Autodesk Inventor part; units mm, degrees
note: some values were not read from the file. Chosen so that the rebuilt part matches the saved one: direction of "Hole2".
(part 17 of 18)
  line L1457 (-0.7456, -14.7218) -> (0.7544, -14.7219)
  line L1458 (0.7544, -14.7219) -> (0.7543, -15.7175)
  line L1459 (0.7543, -15.7175) -> (-0.7457, -15.7174)
  line L1460 (-0.7457, -15.7174) -> (-0.7456, -14.7218)
  line L1461 (0.7544, -14.7219) -> (0.6938, -14.8147)
  line L1462 (-0.7456, -14.7218) -> (-0.6851, -14.8146)
  line L1463 (-0.7457, -15.7174) -> (-0.6885, -15.691)
  line L1464 (0.7543, -15.7175) -> (0.6971, -15.6911)
  line L1465 (3.62, -17.1773) -> (3.8191, -17.1584)
  line L1466 (3.6201, -17.1773) -> (3.62, -17.1773)
  line L1467 (3.8426, -17.4073) -> (3.8427, -17.4073)
  line L1468 (3.8191, -17.1584) -> (3.8426, -17.4073)
  line L1469 (3.7248, -16.1629) -> (3.5257, -16.1817)
  line L1470 (3.7012, -15.914) -> (3.7248, -16.1629)
  line L1471 (3.62, -17.1773) -> (3.5257, -16.1817)
  line L1472 (3.7012, -15.914) -> (5.5927, -15.7349)
  line L1473 (5.7342, -17.2282) -> (3.8426, -17.4073)
  line L1474 (5.8154, -15.9649) -> (5.9097, -16.9604)
  line L1475 (5.5927, -15.7349) -> (5.5928, -15.7349)
  line L1476 (5.8154, -15.9649) -> (5.6163, -15.9837)
  line L1477 (5.6163, -15.9837) -> (5.5927, -15.7349)
  line L1478 (5.8155, -15.9649) -> (5.8154, -15.9649)
  line L1479 (5.7342, -17.2282) -> (5.7106, -16.9793)
  line L1480 (5.7106, -16.9793) -> (5.9097, -16.9604)
  line L1481 (5.9097, -16.9604) -> (5.9098, -16.9604)
  line L1482 (5.7106, -16.9793) -> (5.7107, -16.9793)
  line L1483 (5.7343, -17.2282) -> (5.7342, -17.2282)
  line L1484 (3.9239, -16.144) -> (5.4172, -16.0026)
  line L1485 (5.4172, -16.0026) -> (5.5115, -16.9981)
  line L1486 (5.5115, -16.9981) -> (4.0182, -17.1396)
  line L1487 (4.0182, -17.1396) -> (3.9239, -16.144)
  line L1488 (5.2584, -16.1948) -> (4.1161, -16.303)
  line L1489 (5.4172, -16.0026) -> (5.2584, -16.1948)
  line L1490 (3.9239, -16.144) -> (4.1161, -16.303)
  line L1491 (4.1161, -16.303) -> (4.1772, -16.9474)
  line L1492 (4.0182, -17.1396) -> (4.1772, -16.9474)
  line L1493 (4.1772, -16.9474) -> (5.3194, -16.8392)
  line L1494 (5.5115, -16.9981) -> (5.3194, -16.8392)
  line L1495 (5.3194, -16.8392) -> (5.2584, -16.1948)
  circle A30 centre (4.457, -16.5958) radius 0.1
  line L1496 (4.6323, -16.7299) -> (4.31, -16.7604)
  line L1497 (4.31, -16.7604) -> (4.2817, -16.4617)
  line L1498 (4.2817, -16.4617) -> (4.6041, -16.4312)
  line L1499 (4.6041, -16.4312) -> (4.6323, -16.7299)
  line L1500 (4.6041, -16.4312) -> (4.6324, -16.7299)
  line L1501 (-2.4972, -34.9673) -> (-2.4972, -34.7673)
  line L1502 (-2.4972, -34.7673) -> (-2.2472, -34.7673)
  line L1503 (-3.4972, -34.7672) -> (-3.4972, -34.9672)
  line L1504 (-3.7472, -34.7672) -> (-3.4972, -34.7672)
  line L1505 (-2.4972, -34.9673) -> (-3.4972, -34.9672)
  line L1506 (-3.7472, -34.7672) -> (-3.747, -32.8672)
  line L1507 (-2.247, -32.8673) -> (-2.2472, -34.7673)
  line L1508 (-3.497, -32.6672) -> (-2.497, -32.6673)
  line L1509 (-2.247, -32.8673) -> (-2.497, -32.8673)
  line L1510 (-2.497, -32.8673) -> (-2.497, -32.6673)
  line L1511 (-3.497, -32.6672) -> (-3.497, -32.8672)
  line L1512 (-3.497, -32.8672) -> (-3.747, -32.8672)
  line L1513 (-3.4971, -34.5672) -> (-3.497, -33.0672)
  line L1514 (-3.497, -33.0672) -> (-2.497, -33.0673)
  line L1515 (-2.497, -33.0673) -> (-2.4971, -34.5673)
  line L1516 (-2.4971, -34.5673) -> (-3.4971, -34.5672)
  line L1517 (-3.3207, -33.2435) -> (-3.3208, -34.3909)
  line L1518 (-3.497, -33.0672) -> (-3.3207, -33.2435)
  line L1519 (-3.4971, -34.5672) -> (-3.3208, -34.3909)
  line L1520 (-3.3208, -34.3909) -> (-2.6735, -34.3909)
  line L1521 (-2.4971, -34.5673) -> (-2.6735, -34.3909)
  line L1522 (-2.6735, -34.3909) -> (-2.6734, -33.2436)
  line L1523 (-2.497, -33.0673) -> (-2.6734, -33.2436)
  line L1524 (-2.6734, -33.2436) -> (-3.3207, -33.2435)
  circle A31 centre (-2.9971, -34.0791) radius 0.1
  line L1525 (-2.8471, -33.9172) -> (-2.8471, -34.2411)
  line L1526 (-2.8471, -34.2411) -> (-3.1471, -34.241)
  line L1527 (-3.1471, -34.241) -> (-3.1471, -33.9172)
  line L1528 (-3.1471, -33.9172) -> (-2.8471, -33.9172)
  line L1529 (1.1536, -24.3695) -> (0.9536, -24.3695)
  line L1530 (0.9536, -24.3695) -> (0.9536, -24.1195)
  line L1531 (0.9536, -25.3695) -> (1.1536, -25.3695)
  line L1532 (0.9535, -25.6195) -> (0.9536, -25.3695)
  line L1533 (1.1536, -24.3695) -> (1.1536, -25.3695)
  line L1534 (0.9535, -25.6195) -> (-0.9465, -25.6194)
  line L1535 (-0.9464, -24.1194) -> (0.9536, -24.1195)
  line L1536 (-1.1464, -25.3694) -> (-1.1464, -24.3694)
  line L1537 (-0.9464, -24.1194) -> (-0.9464, -24.3694)
  line L1538 (-0.9464, -24.3694) -> (-1.1464, -24.3694)
  line L1539 (-1.1464, -25.3694) -> (-0.9464, -25.3694)
  line L1540 (-0.9464, -25.3694) -> (-0.9465, -25.6194)
  line L1541 (0.7536, -25.3695) -> (-0.7464, -25.3694)
  line L1542 (-0.7464, -25.3694) -> (-0.7464, -24.3694)
  line L1543 (-0.7464, -24.3694) -> (0.7536, -24.3695)
  line L1544 (0.7536, -24.3695) -> (0.7536, -25.3695)
  line L1545 (-0.5701, -25.1931) -> (0.5772, -25.1932)
  line L1546 (-0.7464, -25.3694) -> (-0.5701, -25.1931)
  line L1547 (0.7536, -25.3695) -> (0.5772, -25.1932)
  line L1548 (0.5772, -25.1932) -> (0.5773, -24.5458)
  line L1549 (0.7536, -24.3695) -> (0.5773, -24.5458)
  line L1550 (0.5773, -24.5458) -> (-0.5701, -24.5457)
  line L1551 (-0.7464, -24.3694) -> (-0.5701, -24.5457)
  line L1552 (-0.5701, -24.5457) -> (-0.5701, -25.1931)
  circle A32 centre (0.2655, -24.8695) radius 0.1
  line L1553 (0.1036, -24.7195) -> (0.4274, -24.7195)
  line L1554 (0.4274, -24.7195) -> (0.4274, -25.0195)
  line L1555 (0.4274, -25.0195) -> (0.1036, -25.0195)
  line L1556 (0.1036, -25.0195) -> (0.1036, -24.7195)
  line L1557 (3.5028, -34.9677) -> (3.5028, -34.7677)
  line L1558 (3.5028, -34.7677) -> (3.7528, -34.7677)
  line L1559 (2.5028, -34.7677) -> (2.5028, -34.9677)
  line L1560 (2.2528, -34.7676) -> (2.5028, -34.7677)
  line L1561 (3.5028, -34.9677) -> (2.5028, -34.9677)
  line L1562 (2.2528, -34.7676) -> (2.253, -32.8676)
  line L1563 (3.753, -32.8677) -> (3.7528, -34.7677)
  line L1564 (2.503, -32.6677) -> (3.503, -32.6677)
  line L1565 (3.753, -32.8677) -> (3.503, -32.8677)
  line L1566 (3.503, -32.8677) -> (3.503, -32.6677)
  line L1567 (2.503, -32.6677) -> (2.503, -32.8677)
  line L1568 (2.503, -32.8677) -> (2.253, -32.8676)
  line L1569 (2.5029, -34.5677) -> (2.503, -33.0677)
  line L1570 (2.503, -33.0677) -> (3.503, -33.0677)
  line L1571 (3.503, -33.0677) -> (3.5029, -34.5677)
  line L1572 (3.5029, -34.5677) -> (2.5029, -34.5677)
  line L1573 (2.6793, -33.244) -> (2.6792, -34.3913)
  line L1574 (2.503, -33.0677) -> (2.6793, -33.244)
  line L1575 (2.5029, -34.5677) -> (2.6792, -34.3913)
  line L1576 (2.6792, -34.3913) -> (3.3265, -34.3914)
  line L1577 (3.5029, -34.5677) -> (3.3265, -34.3914)
  line L1578 (3.3265, -34.3914) -> (3.3266, -33.244)
  line L1579 (3.503, -33.0677) -> (3.3266, -33.244)
  line L1580 (3.3266, -33.244) -> (2.6793, -33.244)
  circle A33 centre (3.0029, -34.0796) radius 0.1
  line L1581 (3.1529, -33.9177) -> (3.1529, -34.2415)
  line L1582 (3.1529, -34.2415) -> (2.8529, -34.2415)
  line L1583 (2.8529, -34.2415) -> (2.8529, -33.9177)
  line L1584 (2.8529, -33.9177) -> (3.1529, -33.9177)
  line L1585 (3.44, -6.9463) -> (3.4399, -7.1453)
  line L1586 (3.4399, -7.1453) -> (3.6899, -7.1453)
  line L1587 (2.4399, -7.1452) -> (2.44, -6.9463)
  line L1588 (2.1899, -7.1452) -> (2.4399, -7.1452)
  line L1589 (3.44, -6.9463) -> (2.44, -6.9463)
  line L1590 (2.1899, -7.1452) -> (2.1898, -8.9031)
  line L1591 (3.6898, -8.9032) -> (3.6899, -7.1453)
  line L1592 (2.4399, -7.3441) -> (2.4398, -8.7045)
  line L1593 (3.4399, -7.3442) -> (2.4399, -7.3441)
  line L1594 (3.4398, -8.7045) -> (3.4399, -7.3442)
  line L1595 (2.4399, -7.3441) -> (2.5999, -7.5976)
  line L1596 (3.4399, -7.3442) -> (3.2799, -7.5977)
  ellipse E659 centre (2.9399, -7.9076) end of major axis (2.8399, -7.9076) minor radius 0.0995
  ellipse E660 centre (2.9399, -7.9128) end of major axis (2.8399, -7.9128) minor radius 0.0995 (2.8399, -7.9128) -> (3.0399, -7.9128) ccw
  line L1597 (3.0399, -7.9076) -> (3.0399, -7.9128)
  line L1598 (2.8399, -7.9076) -> (2.8399, -7.9128)
  line L1599 (3.0899, -8.0739) -> (3.0899, -7.7518)
  line L1600 (3.0899, -8.0844) -> (3.0899, -8.0739)
  line L1601 (3.0899, -7.7518) -> (2.7899, -7.7518)
  line L1602 (2.7899, -7.7518) -> (2.7899, -8.0738)
  line L1603 (2.7899, -8.0844) -> (2.7899, -8.0738)
  line L1604 (2.7899, -8.0738) -> (3.0899, -8.0739)
  line L1605 (7.7865, -8.2785) -> (7.7657, -8.0797)
  line L1606 (7.7657, -8.0797) -> (7.7655, -8.0796)
  line L1607 (7.7655, -8.0796) -> (7.7863, -8.2785)
  line L1608 (7.7863, -8.2785) -> (8.0349, -8.2526)
  line L1609 (8.0349, -8.2526) -> (8.0352, -8.2526)
  line L1610 (6.7917, -8.3825) -> (6.7709, -8.1836)
  line L1611 (6.5431, -8.4085) -> (6.7917, -8.3825)
  line L1612 (8.2175, -9.9969) -> (8.0352, -8.2526)
  line L1613 (7.0103, -10.4712) -> (7.2745, -10.4436)
  line L1614 (7.7655, -8.0796) -> (6.7709, -8.1836)
  line L1615 (6.5431, -8.4085) -> (6.7406, -10.2982)
  line L1616 (7.0101, -10.4711) -> (8.0046, -10.3672)
  line L1617 (8.2325, -10.1423) -> (8.0349, -8.2526)
  line L1618 (6.7409, -10.2983) -> (6.9893, -10.2723)
  line L1619 (6.7406, -10.2982) -> (6.7409, -10.2983)
  line L1620 (6.9893, -10.2722) -> (6.7406, -10.2982)
  line L1621 (7.0101, -10.4711) -> (6.9893, -10.2722)
  line L1622 (7.0103, -10.4712) -> (7.0101, -10.4711)
  line L1623 (7.9839, -10.1682) -> (8.0046, -10.3672)
  line L1624 (8.2325, -10.1423) -> (7.9839, -10.1682)
  line L1625 (6.8125, -8.5814) -> (6.9685, -10.0733)
  line L1626 (7.8071, -8.4775) -> (6.8125, -8.5814)
  line L1627 (7.9631, -9.9693) -> (7.8071, -8.4775)
  line L1628 (6.9685, -10.0733) -> (7.9631, -9.9693)
  line L1629 (7.1257, -9.8797) -> (7.0064, -8.7385)
  line L1630 (6.8125, -8.5814) -> (7.0064, -8.7385)
  line L1631 (6.9685, -10.0733) -> (7.1257, -9.8797)
  line L1632 (7.0064, -8.7385) -> (7.6502, -8.6712)
  line L1633 (7.8071, -8.4775) -> (7.6502, -8.6712)
  line L1634 (7.6502, -8.6712) -> (7.7695, -9.8123)
  line L1635 (7.9631, -9.9693) -> (7.7695, -9.8123)
  line L1636 (7.7695, -9.8123) -> (7.1257, -9.8797)
  circle A34 centre (7.3607, -9.0149) radius 0.1
  line L1637 (7.5267, -9.1604) -> (7.493, -8.8383)
  line L1638 (7.5267, -9.1604) -> (7.5267, -9.1604)
  line L1639 (7.5267, -9.1604) -> (7.4931, -8.8383)
  line L1640 (7.4931, -8.8383) -> (7.493, -8.8383)
  line L1641 (7.493, -8.8383) -> (7.1947, -8.8695)
  line L1642 (7.1947, -8.8695) -> (7.2283, -9.1916)
  line L1643 (7.2284, -9.1916) -> (7.2283, -9.1916)
  line L1644 (7.2283, -9.1916) -> (7.5267, -9.1604)
  line L1645 (7.2284, -9.1916) -> (7.5267, -9.1604)
  line L1646 (3.4398, -8.7045) -> (3.4398, -8.9032)
  line L1647 (3.4398, -8.9032) -> (3.6898, -8.9032)
  line L1648 (2.4398, -8.9031) -> (2.4398, -8.7045)
  line L1649 (2.1898, -8.9031) -> (2.4398, -8.9031)
  line L1650 (3.4397, -10.9527) -> (3.6897, -10.9527)
  line L1651 (3.4397, -10.7904) -> (3.4396, -10.989)
  line L1652 (3.6897, -10.7904) -> (3.4397, -10.7904)
  line L1653 (3.4396, -10.989) -> (3.4396, -11.1513)
  line L1654 (3.6897, -10.9527) -> (3.6897, -10.7904)
  line L1655 (2.4396, -11.1513) -> (3.4396, -11.1513)
  line L1656 (3.4398, -8.7045) -> (2.4398, -8.7045)
  line L1657 (2.1898, -8.9031) -> (2.1897, -10.7903)
  line L1658 (2.4396, -10.989) -> (3.4396, -10.989)
  line L1659 (3.6897, -10.7904) -> (3.6898, -8.9032)
  line L1660 (2.1897, -10.9526) -> (2.4397, -10.9526)
  line L1661 (2.1897, -10.7903) -> (2.1897, -10.9526)
  line L1662 (2.4397, -10.7903) -> (2.1897, -10.7903)
  line L1663 (2.4396, -10.989) -> (2.4397, -10.7903)
  line L1664 (2.4396, -11.1513) -> (2.4396, -10.989)
  line L1665 (2.4398, -9.1018) -> (2.4397, -10.5917)
  line L1666 (3.4398, -9.1019) -> (2.4398, -9.1018)
  line L1667 (3.4397, -10.5917) -> (3.4398, -9.1019)
  line L1668 (2.4397, -10.5917) -> (3.4397, -10.5917)
  line L1669 (2.616, -10.5325) -> (2.6161, -9.3928)
  line L1670 (2.4398, -9.1018) -> (2.6161, -9.3928)
  line L1671 (2.4397, -10.5917) -> (2.616, -10.5325)
  line L1672 (2.6161, -9.3928) -> (3.2634, -9.3929)
  line L1673 (3.4398, -9.1019) -> (3.2634, -9.3929)
  line L1674 (3.2634, -9.3929) -> (3.2634, -10.5325)
  line L1675 (3.4397, -10.5917) -> (3.2634, -10.5325)
  line L1676 (3.2634, -10.5325) -> (2.616, -10.5325)
  ellipse E661 centre (2.9397, -9.6736) end of major axis (2.8397, -9.6735) minor radius 0.0993
  ellipse E662 centre (2.9397, -9.6793) end of major axis (2.8397, -9.6793) minor radius 0.0993 (2.8397, -9.6793) -> (3.0397, -9.6794) ccw
  line L1677 (3.0397, -9.6736) -> (3.0397, -9.6794)
  line L1678 (2.8397, -9.6735) -> (2.8397, -9.6793)
  line L1679 (3.0897, -9.8402) -> (3.0898, -9.5185)
  line L1680 (3.0897, -9.8634) -> (3.0897, -9.8402)
  line L1681 (3.0898, -9.5185) -> (2.7898, -9.5185)
  line L1682 (2.7898, -9.5185) -> (2.7897, -9.8402)
  line L1683 (2.7897, -9.8633) -> (2.7897, -9.8402)
  line L1684 (2.7897, -9.8402) -> (3.0897, -9.8402)
  line L1685 (2.7897, -9.8633) -> (3.0897, -9.8634)
  line L1686 (8.4774, -9.9666) -> (8.4772, -9.9665)
  line L1687 (8.4772, -9.9665) -> (8.5004, -10.1652)
  line L1688 (8.5004, -10.1652) -> (8.7488, -10.1362)
  line L1689 (8.7488, -10.1362) -> (8.7489, -10.1363)
  line L1690 (8.9692, -12.0234) -> (8.7489, -10.1363)
  line L1691 (8.7164, -12.2543) -> (8.7441, -12.2511)
  line L1692 (8.4772, -9.9665) -> (8.2173, -9.9969)
  line L1693 (7.2744, -10.4435) -> (7.4792, -12.1973)
  line L1694 (7.7507, -12.367) -> (8.744, -12.251)
  line L1695 (8.9691, -12.0234) -> (8.7488, -10.1362)
  line L1696 (8.7488, -12.0492) -> (8.9692, -12.0234)
  line L1697 (8.7441, -12.2511) -> (8.7328, -12.1544)
  line L1698 (8.7208, -12.0524) -> (8.744, -12.251)
  line L1699 (8.9691, -12.0234) -> (8.7208, -12.0524)
  line L1700 (8.7208, -12.0524) -> (8.7209, -12.0524)
  line L1701 (8.744, -12.251) -> (8.7441, -12.2511)
  line L1702 (8.9692, -12.0234) -> (8.9691, -12.0234)
  line L1703 (7.4792, -12.1973) -> (7.4794, -12.1974)
  line L1704 (7.7275, -12.1683) -> (7.4792, -12.1973)
  line L1705 (7.7507, -12.367) -> (7.7275, -12.1683)
  line L1706 (7.7509, -12.3671) -> (7.7507, -12.367)
  line L1707 (7.5304, -10.4798) -> (7.7043, -11.9697)
  line L1708 (8.5236, -10.3638) -> (7.5304, -10.4798)
  line L1709 (8.6976, -11.8537) -> (8.5236, -10.3638)
  line L1710 (7.7043, -11.9697) -> (8.6976, -11.8537)
  line L1711 (7.8591, -11.7741) -> (7.7261, -10.6345)
  line L1712 (7.5304, -10.4798) -> (7.7261, -10.6345)
  line L1713 (7.7043, -11.9697) -> (7.8591, -11.7741)
  line L1714 (7.7261, -10.6345) -> (8.369, -10.5595)
  line L1715 (8.5236, -10.3638) -> (8.369, -10.5595)
  line L1716 (8.369, -10.5595) -> (8.5021, -11.6991)
  line L1717 (8.6976, -11.8537) -> (8.5021, -11.6991)
  line L1718 (8.5021, -11.6991) -> (7.8591, -11.7741)
  circle A35 centre (8.0837, -10.9067) radius 0.1
  line L1719 (8.2515, -11.0501) -> (8.2139, -10.7284)
  line L1720 (8.2515, -11.0501) -> (8.2515, -11.0501)
  line L1721 (8.2515, -11.0501) -> (8.2139, -10.7285)
  line L1722 (8.2139, -10.7285) -> (8.2139, -10.7284)
  line L1723 (8.2139, -10.7284) -> (7.9159, -10.7632)
  line L1724 (7.9159, -10.7632) -> (7.9535, -11.0849)
  line L1725 (7.9535, -11.0849) -> (7.9535, -11.0849)
  line L1726 (7.9535, -11.0849) -> (8.2515, -11.0501)
  line L1727 (7.9535, -11.0849) -> (8.2515, -11.0501)
  line L1728 (3.4401, -5.1401) -> (3.4401, -5.3392)
  line L1729 (3.4401, -5.3392) -> (3.6901, -5.3392)
  line L1730 (2.4401, -5.3391) -> (2.4401, -5.14)
  line L1731 (2.1901, -5.3391) -> (2.4401, -5.3391)
  line L1732 (3.4401, -5.1401) -> (2.4401, -5.14)
  line L1733 (2.1901, -5.3391) -> (2.1899, -7.1452)
  line L1734 (3.6899, -7.1453) -> (3.6901, -5.3392)
  line L1735 (2.4401, -5.5382) -> (2.44, -6.9463)
  line L1736 (3.4401, -5.5383) -> (2.4401, -5.5382)
  line L1737 (3.44, -6.9463) -> (3.4401, -5.5383)
  line L1738 (2.6163, -6.2888) -> (2.6164, -5.8081)
  line L1739 (2.4401, -5.5382) -> (2.6164, -5.8081)
  line L1740 (2.6164, -5.8081) -> (3.2637, -5.8081)
  line L1741 (3.4401, -5.5383) -> (3.2637, -5.8081)
  line L1742 (3.2637, -5.8081) -> (3.2637, -6.2888)
  ellipse E663 centre (2.94, -6.0949) end of major axis (2.84, -6.0949) minor radius 0.0996
  ellipse E664 centre (2.94, -6.0996) end of major axis (2.84, -6.0996) minor radius 0.0996 (2.84, -6.0996) -> (3.04, -6.0996) ccw
  line L1743 (3.04, -6.0949) -> (3.04, -6.0996)
  line L1744 (2.84, -6.0949) -> (2.84, -6.0996)
  line L1745 (3.09, -6.2608) -> (3.09, -5.9384)
  line L1746 (3.09, -6.2797) -> (3.09, -6.2608)
  line L1747 (3.09, -5.9384) -> (2.79, -5.9384)
  line L1748 (2.79, -5.9384) -> (2.79, -6.2608)
  line L1749 (2.79, -6.2797) -> (2.79, -6.2608)
  line L1750 (2.79, -6.2608) -> (3.09, -6.2608)
  line L1751 (2.79, -6.2797) -> (3.09, -6.2797)
  line L1752 (7.2017, -6.3664) -> (7.1828, -6.1673)
  line L1753 (7.1828, -6.1673) -> (7.1827, -6.1673)
  line L1754 (7.1827, -6.1673) -> (7.2016, -6.3664)
  line L1755 (7.2016, -6.3664) -> (7.4505, -6.3429)
  line L1756 (7.4505, -6.3429) -> (7.4506, -6.3429)
  line L1757 (6.206, -6.4607) -> (6.1872, -6.2616)
  line L1758 (5.9572, -6.4843) -> (6.206, -6.4607)
  line L1759 (7.4714, -6.563) -> (7.4506, -6.3429)
  line L1760 (7.1827, -6.1673) -> (6.1872, -6.2616)
  line L1761 (5.9572, -6.4843) -> (6.1363, -8.3758)
  line L1762 (6.404, -8.5514) -> (6.5565, -8.5369)
  line L1763 (7.6164, -8.0952) -> (7.4505, -6.3429)
  line L1764 (6.1363, -8.3758) -> (6.1364, -8.3758)
  line L1765 (6.3852, -8.3522) -> (6.1363, -8.3758)
  line L1766 (6.404, -8.5514) -> (6.3852, -8.3522)
  line L1767 (6.4041, -8.5514) -> (6.404, -8.5514)
  line L1768 (6.2249, -6.6598) -> (6.3663, -8.1531)
  line L1769 (7.2204, -6.5655) -> (6.2249, -6.6598)
  line L1770 (7.3619, -8.0589) -> (7.2204, -6.5655)
  line L1771 (6.3663, -8.1531) -> (7.3619, -8.0589)
  line L1772 (6.5253, -7.961) -> (6.4171, -6.8187)
  line L1773 (6.2249, -6.6598) -> (6.4171, -6.8187)
  line L1774 (6.3663, -8.1531) -> (6.5253, -7.961)
  line L1775 (6.4171, -6.8187) -> (7.0616, -6.7577)
  line L1776 (7.2204, -6.5655) -> (7.0616, -6.7577)
  line L1777 (7.0616, -6.7577) -> (7.1698, -7.8999)
  line L1778 (7.3619, -8.0589) -> (7.1698, -7.8999)
  line L1779 (7.1698, -7.8999) -> (6.5253, -7.961)
  circle A36 centre (6.7687, -7.0986) radius 0.1
  line L1780 (6.9333, -7.2456) -> (6.9028, -6.9233)
  line L1781 (6.9334, -7.2456) -> (6.9028, -6.9233)
  line L1782 (6.9028, -6.9233) -> (6.6042, -6.9515)
  line L1783 (6.6042, -6.9515) -> (6.6347, -7.2739)
  line L1784 (6.6347, -7.2739) -> (6.9333, -7.2456)
  ellipse E665 centre (-10.5208, -10.2386) end of major axis (-11.7192, -10.2991) minor radius 0.2145 (-9.7641, -10.035) -> (-11.6973, -10.337) ccw
  ellipse E666 centre (-10.5108, -10.4351) end of major axis (-11.5096, -10.4855) minor radius 0.1787 (-9.9788, -10.2576) -> (-11.2971, -10.5839) ccw
  line L1785 (-11.4913, -10.5171) -> (-11.6973, -10.337)
  ellipse E667 centre (-10.5108, -10.4351) end of major axis (-11.2599, -10.4729) minor radius 0.134 (-10.2354, -10.2968) -> (-11.0503, -10.5546) ccw
  line L1786 (-11.7192, -10.2991) -> (-11.7621, -9.4506)
  ellipse E668 centre (10.5302, -10.2402) end of major axis (11.7286, -10.3008) minor radius 0.2145 (11.7067, -10.3387) -> (9.7736, -10.0365) ccw
  ellipse E669 centre (10.5202, -10.4367) end of major axis (11.5189, -10.4873) minor radius 0.1787 (11.3065, -10.5856) -> (9.9882, -10.2592) ccw
  line L1787 (11.5007, -10.5188) -> (11.7067, -10.3387)
  ellipse E670 centre (10.5202, -10.4367) end of major axis (11.2693, -10.4746) minor radius 0.134 (11.0597, -10.5562) -> (10.2448, -10.2984) ccw
  line L1788 (11.7286, -10.3008) -> (11.7716, -9.4523)
  ellipse E671 centre (0.0058, 4.4476) end of major axis (-0.5606, 4.4476) minor radius 0.5639 (0.3748, 4.0197) -> (-0.3632, 4.0198) ccw
  line L1789 (-0.1078, 4.8404) -> (0.2908, 4.7419)
  line L1790 (0.2908, 4.7419) -> (0.4043, 4.3491)
  line L1791 (0.4043, 4.3491) -> (0.1426, 4.0787)
  line L1792 (-0.109, 4.1112) -> (-0.2791, 4.1533)
  line L1793 (-0.2791, 4.1533) -> (-0.3927, 4.5461)
  line L1794 (-0.3927, 4.5461) -> (-0.1078, 4.8404)
  line L1795 (0.2908, 4.7419) -> (0.2908, 4.6522)
  line L1796 (-0.1078, 4.7512) -> (-0.1078, 4.8404)
  spline S53 degree 3 poles (-11.5926, -40.3717) (-11.5879, -40.3723) (-11.5775, -40.3737) (-11.5629, -40.3833) (-11.5483, -40.3978) (-11.534, -40.4182) (-11.5201, -40.4438) (-11.5015, -40.4866) (-11.4857, -40.5356) (-11.472, -40.5901) (-11.4587, -40.6545) (-11.4454, -40.7428) (-11.436, -40.854) (-11.4327, -40.9686) (-11.436, -41.0832) (-11.4454, -41.1944) (-11.4587, -41.2827) (-11.4721, -41.3471) (-11.4857, -41.4016) (-11.5015, -41.4506) (-11.5202, -41.4934) (-11.534, -41.519) (-11.5484, -41.5393) (-11.563, -41.5539) (-11.5776, -41.5635) (-11.588, -41.5649) (-11.5927, -41.5655) knots 0 0 0 0 0.011067 0.024078 0.039928 0.05914 0.081934 0.10802 0.168059 0.202015 0.239296 0.321668 0.410563 0.5 0.589437 0.678332 0.760704 0.797985 0.831941 0.89198 0.918066 0.94086 0.960072 0.975922 0.988933 1 1 1 1
  spline S54 degree 3 poles (-11.5927, -41.5655) (-11.5974, -41.5649) (-11.6074, -41.5636) (-11.6213, -41.5539) (-11.6345, -41.5393) (-11.6471, -41.5189) (-11.6587, -41.4933) (-11.6738, -41.4504) (-11.6859, -41.4014) (-11.696, -41.347) (-11.7056, -41.2825) (-11.7148, -41.1942) (-11.7211, -41.0831) (-11.7233, -40.9686) (-11.7211, -40.8541) (-11.7148, -40.743) (-11.7055, -40.6546) (-11.6959, -40.5902) (-11.6858, -40.5358) (-11.6737, -40.4868) (-11.6586, -40.4439) (-11.647, -40.4182) (-11.6345, -40.3979) (-11.6212, -40.3833) (-11.6073, -40.3736) (-11.5973, -40.3723) (-11.5926, -40.3717) knots 0 0 0 0 0.010997 0.023628 0.038954 0.057614 0.079908 0.105595 0.165209 0.199149 0.236543 0.319515 0.409403 0.5 0.590597 0.680485 0.763457 0.800851 0.834791 0.894405 0.920092 0.942386 0.961046 0.976372 0.989003 1 1 1 1
  spline S55 degree 3 poles (11.5974, -41.5672) (11.5926, -41.5666) (11.5823, -41.5653) (11.5676, -41.5556) (11.5531, -41.5411) (11.5387, -41.5208) (11.5248, -41.4951) (11.5062, -41.4523) (11.4904, -41.4033) (11.4768, -41.3488) (11.4634, -41.2844) (11.4501, -41.1961) (11.4407, -41.0849) (11.4374, -40.9703) (11.4408, -40.8557) (11.4501, -40.7445) (11.4635, -40.6562) (11.4768, -40.5918) (11.4905, -40.5374) (11.5063, -40.4883) (11.5249, -40.4456) (11.5388, -40.4199) (11.5531, -40.3996) (11.5677, -40.3851) (11.5824, -40.3754) (11.5927, -40.3741) (11.5974, -40.3734) knots 0 0 0 0 0.011067 0.024078 0.039928 0.05914 0.081934 0.10802 0.168059 0.202015 0.239296 0.321668 0.410563 0.5 0.589437 0.678332 0.760704 0.797985 0.831941 0.89198 0.918066 0.94086 0.960072 0.975922 0.988933 1 1 1 1
  spline S56 degree 3 poles (11.5974, -40.3734) (11.6021, -40.3741) (11.6121, -40.3754) (11.626, -40.385) (11.6393, -40.3996) (11.6518, -40.42) (11.6634, -40.4457) (11.6786, -40.4886) (11.6906, -40.5376) (11.7007, -40.5919) (11.7103, -40.6564) (11.7196, -40.7448) (11.7259, -40.8559) (11.7281, -40.9704) (11.7259, -41.0848) (11.7195, -41.1959) (11.7103, -41.2843) (11.7006, -41.3488) (11.6906, -41.4031) (11.6785, -41.4521) (11.6634, -41.495) (11.6517, -41.5207) (11.6392, -41.541) (11.626, -41.5556) (11.612, -41.5653) (11.602, -41.5666) (11.5974, -41.5672) knots 0 0 0 0 0.010997 0.023628 0.038954 0.057614 0.079908 0.105595 0.165209 0.199149 0.236543 0.319515 0.409403 0.5 0.590597 0.680485 0.763457 0.800851 0.834791 0.894405 0.920092 0.942386 0.961046 0.976372 0.989003 1 1 1 1
  line L1797 (-4.2111, -43.3771) -> (-4.2111, -43.4691)
  line L1798 (-9.1521, -43.4688) -> (-9.152, -42.8688)
  line L1799 (-4.2111, -43.4691) -> (-9.1521, -43.4688)
  line L1800 (4.2154, -43.4698) -> (4.2154, -43.3778)
  line L1801 (9.1564, -43.4702) -> (4.2154, -43.4698)
  line L1802 (9.1565, -42.8702) -> (9.1564, -43.4702)
  line L1803 (-3.9978, -42.8692) -> (-9.152, -42.8688)
  line L1804 (9.1565, -42.8702) -> (4.0022, -42.8698)
  line L1805 (11.9522, -43.4704) -> (9.1564, -43.4702)
  line L1806 (-9.1521, -43.4688) -> (-11.9478, -43.4686)
  line L1807 (4.0026, -38.4698) -> (11.9526, -38.4704)
  line L1808 (-11.9474, -38.4686) -> (-3.9974, -38.4692)
  line L1809 (-11.9478, -43.4686) -> (-11.9474, -38.4686)
  line L1810 (11.9522, -43.4704) -> (11.9526, -38.4704)
  line L1811 (4.2154, -43.4698) -> (3.9056, -43.4698)
  line L1812 (3.9056, -43.4698) -> (3.9056, -43.3778)
  line L1813 (3.9056, -43.4698) -> (-4.2111, -43.4691)
  line L1814 (-9.079, -28.4688) -> (-3.3218, -28.4692)
  line L1815 (3.3285, -28.4697) -> (9.0857, -28.4702)
  line L1816 (10.6536, -28.4703) -> (11.2166, -28.4703)
  line L1817 (-11.21, -28.4686) -> (-10.6469, -28.4687)
  line L1818 (11.2159, -38.4703) -> (11.2166, -28.4703)
  line L1819 (-11.21, -28.4686) -> (-11.2107, -38.4686)
  spline S57 degree 3 poles (-8.765, -35.8678) (-8.7648, -35.7576) (-8.7613, -35.5337) (-8.7432, -35.2012) (-8.7131, -34.928) (-8.6797, -34.7387) (-8.6452, -34.6465) (-8.6218, -34.584) (-8.5726, -34.5816) (-8.545, -34.6216) (-8.5101, -34.7022) (-8.473, -34.8884) (-8.4416, -35.1618) (-8.4237, -35.4932) (-8.4193, -35.8266) (-8.4269, -36.1595) (-8.4469, -36.4934) (-8.4788, -36.7654) (-8.5146, -36.9551) (-8.547, -37.0463) (-8.5709, -37.112) (-8.6202, -37.1122) (-8.6466, -37.0707) (-8.6773, -36.9901) (-8.7144, -36.8043) (-8.7436, -36.5319) (-8.7612, -36.1997) (-8.7653, -35.9771) (-8.765, -35.8678) knots 0 0 0 0 0.063707 0.129495 0.191912 0.223688 0.23829 0.25135 0.256604 0.263018 0.277149 0.308538 0.37104 0.436878 0.500023 0.563695 0.629383 0.692836 0.723161 0.738573 0.75181 0.756962 0.76326 0.777952 0.808043 0.871314 0.936843 1 1 1 1
  spline S58 degree 3 poles (-10.9612, -35.7861) (-10.9606, -35.5634) (-10.9502, -35.2395) (-10.9501, -34.8431) (-10.9123, -34.685) (-10.9216, -34.5912) (-10.8849, -34.5812) (-10.8742, -34.6616) (-10.8557, -34.7489) (-10.8407, -34.9692) (-10.8272, -35.2391) (-10.8199, -35.5729) (-10.8159, -36.0193) (-10.8316, -36.4522) (-10.8351, -36.8493) (-10.8749, -37.0082) (-10.8656, -37.1028) (-10.9029, -37.1132) (-10.9115, -37.0308) (-10.9295, -36.9438) (-10.9417, -36.7227) (-10.9578, -36.3453) (-10.9618, -36.0091) (-10.9612, -35.7861) knots 0 0 0 0 0.131392 0.195062 0.224866 0.236537 0.238771 0.243638 0.272647 0.302988 0.368078 0.435032 0.499113 0.631038 0.694715 0.724747 0.73665 0.738894 0.743873 0.773079 0.803452 0.868455 1 1 1 1
  spline S59 degree 3 poles (8.4267, -35.7875) (8.427, -35.6772) (8.4301, -35.4526) (8.452, -35.1237) (8.4814, -34.8431) (8.5289, -34.6765) (8.565, -34.5846) (8.614, -34.5834) (8.6573, -34.6455) (8.6878, -34.7566) (8.7246, -34.9687) (8.7518, -35.2448) (8.7681, -35.5762) (8.7723, -35.9095) (8.7653, -36.2428) (8.7457, -36.572) (8.7151, -36.8516) (8.6714, -37.0192) (8.6391, -37.1111) (8.5896, -37.1148) (8.546, -37.0492) (8.5183, -36.9401) (8.4769, -36.7277) (8.4498, -36.4528) (8.4307, -36.1196) (8.4264, -35.8968) (8.4267, -35.7875) knots 0 0 0 0 0.063774 0.129476 0.191917 0.222516 0.235727 0.240982 0.247121 0.27643 0.308417 0.371002 0.43691 0.500019 0.563738 0.62925 0.691939 0.722123 0.735387 0.74054 0.746943 0.777028 0.807219 0.871188 0.93687 1 1 1 1
  line L1820 (9.0857, -28.4702) -> (10.6536, -28.4703)
  line L1821 (-10.6469, -28.4687) -> (-9.079, -28.4688)
  spline S60 degree 3 poles (10.824, -35.8693) (10.8247, -35.6454) (10.8266, -35.3114) (10.851, -34.9324) (10.8597, -34.7394) (10.8833, -34.6541) (10.8768, -34.5883) (10.9141, -34.585) (10.9175, -34.6303) (10.937, -34.7026) (10.9458, -34.8943) (10.9603, -35.163) (10.9658, -35.4953) (10.9676, -35.9408) (10.9641, -36.3865) (10.9431, -36.7634) (10.9356, -36.9581) (10.9141, -37.0404) (10.9216, -37.1121) (10.884, -37.1112) (10.8809, -37.0656) (10.8614, -36.9927) (10.8498, -36.8019) (10.8272, -36.4259) (10.8233, -36.0918) (10.824, -35.8693) knots 0 0 0 0 0.132092 0.195475 0.227359 0.241584 0.252969 0.255186 0.260256 0.27356 0.304855 0.368241 0.435353 0.499807 0.631725 0.696074 0.726444 0.741485 0.752997 0.755195 0.760334 0.774394 0.8045 0.86873 1 1 1 1
  line L1822 (4.0031, -30.9398) -> (2.0037, -23.6196)
  line L1823 (-1.9963, -23.6193) -> (-3.9969, -30.9392)
  line L1824 (4.0023, -42.3618) -> (4.0031, -30.9398)
  line L1825 (-3.9977, -42.3612) -> (-3.9969, -30.9392)
  line L1826 (2.0037, -23.6196) -> (-1.9963, -23.6193)
  line L1827 (4.0023, -42.3618) -> (4.0022, -43.3778)
  line L1828 (-3.9977, -42.3612) -> (-3.9978, -43.3772)
  line L1829 (4.0022, -43.3778) -> (-3.9978, -43.3772)
  line L1830 (-8.1228, -43.3768) -> (-8.2976, -43.3768)
  line L1831 (-8.1227, -42.8688) -> (-8.1228, -43.3768)
  line L1832 (-4.4204, -43.3771) -> (-8.1228, -43.3768)
  line L1833 (-4.4204, -43.3771) -> (-3.9978, -43.3772)
  line L1834 (4.0022, -43.3778) -> (4.4247, -43.3778)
  line L1835 (8.1272, -43.3781) -> (4.4247, -43.3778)
  line L1836 (8.1272, -42.8701) -> (8.1272, -43.3781)
  line L1837 (8.302, -43.3781) -> (8.1272, -43.3781)
  line L1838 (-8.2976, -42.8688) -> (-8.2976, -43.3768)
  line L1839 (8.3021, -42.8701) -> (8.302, -43.3781)
  line L1840 (-10.998, -46.4686) -> (11.002, -46.4703)
  line L1841 (-11.0006, -79.4686) -> (10.9994, -79.4703)
  line L1842 (-11.0006, -79.4686) -> (-10.998, -46.4686)
  line L1843 (10.9994, -79.4703) -> (11.002, -46.4703)
  line L1844 (-9.3965, -46.4687) -> (-9.3963, -43.4687)
  line L1845 (-7.2965, -46.4689) -> (-7.2963, -43.4689)
  line L1846 (-1.048, -46.4694) -> (-1.0478, -43.4694)
  line L1847 (1.052, -46.4695) -> (1.0522, -43.4695)
  line L1848 (7.3004, -46.47) -> (7.3007, -43.47)
  line L1849 (9.4004, -46.4702) -> (9.4007, -43.4702)
  spline S61 degree 3 poles (-9.494, -108.2993) (-9.353, -108.713) (-9.0666, -109.5532) (-8.6901, -110.8592) (-8.3692, -112.2354) (-8.1311, -113.648) (-7.9812, -115.0492) (-7.9058, -116.3975) (-7.8805, -117.6999) (-7.8805, -118.5546) (-7.8805, -118.9769) knots 0 0 0 0 0.131107 0.266278 0.407581 0.554823 0.69573 0.830104 0.959816 1.086502 1.086502 1.086502 1.086502
  spline S62 degree 3 poles (-11.494, -103.9948) (-11.494, -103.9946) (-11.494, -103.9937) (-11.494, -103.9918) (-11.494, -103.9886) (-11.494, -103.9842) (-11.494, -103.9785) (-11.494, -103.9716) (-11.494, -103.9634) (-11.494, -103.954) (-11.494, -103.9434) (-11.494, -103.9315) (-11.494, -103.9184) (-11.494, -103.9041) (-11.494, -103.8886) (-11.494, -103.872) (-11.494, -103.8542) (-11.494, -103.842) (-11.494, -103.8357) knots 0 0 0 0 0.003987 0.015957 0.035891 0.063749 0.099497 0.143102 0.194528 0.253743 0.320712 0.395401 0.477746 0.567575 0.664794 0.769325 0.881087 1 1 1 1
  spline S63 degree 3 poles (-11.494, -103.8357) (-11.3405, -104.2193) (-11.0359, -104.9806) (-10.3609, -106.4655) (-9.8405, -107.5662) (-9.494, -108.2993) knots 0 0 0 0 0.253343 0.502767 1 1 1 1
  spline S64 degree 3 poles (6.82, -107.936) (6.6704, -108.3625) (6.3662, -109.2297) (5.9601, -110.5782) (5.6105, -112.0026) (5.3492, -113.4664) (5.1842, -114.918) (5.101, -116.3127) (5.0732, -117.6582) (5.0731, -118.5408) (5.0731, -118.9769) knots 0 0 0 0 0.135587 0.27568 0.422315 0.575323 0.72143 0.860365 0.994299 1.125132 1.125132 1.125132 1.125132
  line L1850 (4.82, -103.423) -> (4.82, -118.9769)
  line L1851 (5.0731, -118.9769) -> (4.82, -118.9769)
  line L1852 (4.82, -118.9769) -> (2.82, -118.9769)
  spline S65 degree 3 poles (2.82, -118.9769) (2.82, -118.0946) (2.82, -116.7501) (2.82, -114.9219) (2.82, -113.4739) (2.82, -112.013) (2.82, -110.5885) (2.82, -109.2384) (2.82, -108.3634) (2.82, -107.9357) knots 0 0 0 0 0.264693 0.403339 0.548464 0.699098 0.841605 0.975818 1.104119 1.104119 1.104119 1.104119
  spline S66 degree 3 poles (2.82, -107.9357) (3.1728, -107.1995) (3.7031, -106.0925) (4.2838, -104.7796) (4.5984, -104.0118) (4.7458, -103.6201) (4.82, -103.423) knots 0 0 0 0 0.495968 0.745691 0.872094 1 1 1 1
  spline S67 degree 3 poles (4.82, -103.423) (4.9016, -103.448) (5.0643, -103.4979) (5.3143, -103.5485) (5.5664, -103.5801) (5.8201, -103.5905) (6.0736, -103.5801) (6.3259, -103.5486) (6.5758, -103.498) (6.7385, -103.4481) (6.82, -103.4232) knots 0 0 0 0 0.125726 0.250746 0.375528 0.500005 0.624584 0.749245 0.874433 1 1 1 1
  spline S68 degree 3 poles (6.82, -103.4232) (6.82, -103.8125) (6.82, -104.5782) (6.82, -106.0825) (6.82, -107.1974) (6.82, -107.936) knots 0 0 0 0 0.25882 0.509015 1 1 1 1
  line L1853 (-9.494, -92.4769) -> (-9.494, -108.2993)
  line L1854 (-9.494, -92.4769) -> (-7.494, -92.4769)
  line L1855 (-7.494, -92.4769) -> (-7.494, -118.9769)
  line L1856 (-11.494, -92.4769) -> (-11.494, -103.8357)
  line L1857 (-11.494, -92.4769) -> (-9.494, -92.4769)
  line L1858 (2.82, -92.4769) -> (2.82, -107.9357)
  line L1859 (2.82, -92.4769) -> (4.82, -92.4769)
  line L1860 (4.82, -92.4769) -> (4.82, -103.423)
  line L1861 (4.82, -92.4769) -> (6.82, -92.4769)
  line L1862 (6.82, -92.4769) -> (6.82, -103.4232)
  line L1863 (2.074, -92.4769) -> (2.074, -118.9769)
  line L1864 (2.074, -92.4769) -> (2.82, -92.4769)
  line L1865 (4.074, -92.4769) -> (4.074, -118.9769)
  line L1866 (6.074, -92.4769) -> (6.074, -108.4438)
  spline S69 degree 3 poles (4.4528, -118.9769) (4.4528, -118.5603) (4.4528, -117.7174) (4.4782, -116.4329) (4.5541, -115.1033) (4.7048, -113.7212) (4.9442, -112.3272) (5.2667, -110.9689) (5.6447, -109.6801) (5.9324, -108.8516) (6.074, -108.4438) knots 0 0 0 0 0.124973 0.252876 0.385371 0.524366 0.669742 0.809378 0.942972 1.072465 1.072465 1.072465 1.072465
  spline S70 degree 3 poles (6.074, -103.6797) (5.9878, -103.6852) (5.8156, -103.6962) (5.5566, -103.6853) (5.299, -103.6544) (5.0441, -103.6021) (4.7929, -103.5297) (4.5468, -103.4378) (4.3057, -103.3289) (4.1514, -103.2428) (4.074, -103.1996) knots 0 0 0 0 0.12386 0.247576 0.371585 0.495852 0.620749 0.746432 0.87277 1 1 1 1
  spline S71 degree 3 poles (4.074, -103.1996) (4.0019, -103.3856) (3.8585, -103.7557) (3.5507, -104.4815) (3.1412, -105.3699) (2.6176, -106.4173) (2.2554, -107.1076) (2.074, -107.4533) knots 0 0 0 0 0.127199 0.253182 0.502754 0.751027 1 1 1 1
  line L1867 (12, -89.9769) -> (-12, -89.9769)
  line L1868 (9.484, 23.984) -> (-9.484, 23.984)
  line L1869 (9.9707, 23.5986) -> (-9.9707, 23.5986)
  spline S72 degree 3 poles (-10.984, 5) (-10.8382, 5.1991) (-10.5443, 5.6007) (-9.8968, 6.3741) (-9.2177, 7.1334) (-8.5715, 7.9299) (-8.2022, 8.4588) (-7.9409, 8.9054) (-7.7649, 9.2552) (-7.6085, 9.6198) (-7.5257, 9.8725) (-7.484, 10) knots 0 0 0 0 0.074013 0.149267 0.302447 0.379596 0.456855 0.495662 0.534746 0.574288 0.614507 0.614507 0.614507 0.614507
  spline S73 degree 3 poles (10.984, 5) (10.8382, 5.1991) (10.5443, 5.6007) (9.8968, 6.3741) (9.2177, 7.1334) (8.5715, 7.9299) (8.2022, 8.4588) (7.9409, 8.9054) (7.7649, 9.2552) (7.6085, 9.6198) (7.5257, 9.8725) (7.484, 10) knots 0 0 0 0 0.074013 0.149267 0.302447 0.379596 0.456855 0.495662 0.534746 0.574288 0.614507 0.614507 0.614507 0.614507
  spline S74 degree 3 poles (-12.5, 0) (-12.4969, 0.2228) (-12.4906, 0.6682) (-12.4311, 1.3327) (-12.3255, 1.9886) (-12.166, 2.6306) (-11.9514, 3.2549) (-11.6807, 3.8588) (-11.3597, 4.4438) (-11.1098, 4.8138) (-10.984, 5) knots 0 0 0 0 0.066832 0.133581 0.19996 0.265954 0.331772 0.397749 0.464268 0.531651 0.531651 0.531651 0.531651
  spline S75 degree 3 poles (12.5, 0) (12.4969, 0.2228) (12.4906, 0.6682) (12.4311, 1.3327) (12.3255, 1.9886) (12.166, 2.6306) (11.9514, 3.2549) (11.6807, 3.8588) (11.3597, 4.4438) (11.1098, 4.8138) (10.984, 5) knots 0 0 0 0 0.066832 0.133581 0.19996 0.265954 0.331772 0.397749 0.464268 0.531651 0.531651 0.531651 0.531651
  arc A37 (9.9707, 23.5986) -> (9.484, 23.984) centre (9.484, 23.484) ccw
  arc A38 (-9.484, 23.984) -> (-9.9707, 23.5986) centre (-9.484, 23.484) ccw
  spline S76 degree 3 poles (-7.484, 10) (-7.4299, 10.2009) (-7.319, 10.612) (-7.2347, 11.2639) (-7.2073, 11.9563) (-7.2448, 12.6916) (-7.3412, 13.4681) (-7.4928, 14.2848) (-7.6958, 15.1387) (-8.0294, 16.3449) (-8.5255, 17.9031) (-9.1497, 19.7993) (-9.6091, 21.4019) (-9.8773, 22.671) (-9.94, 23.2943) (-9.9707, 23.5986) knots 0 0 0 0 0.062347 0.127633 0.196641 0.270049 0.348203 0.431234 0.519115 0.611423 0.806629 1.009594 1.210352 1.306485 1.398176 1.398176 1.398176 1.398176
  spline S77 degree 3 poles (7.484, 10) (7.4299, 10.2009) (7.319, 10.612) (7.2347, 11.2639) (7.2073, 11.9563) (7.2448, 12.6916) (7.3412, 13.4681) (7.4928, 14.2848) (7.6958, 15.1387) (8.0294, 16.3449) (8.5255, 17.9031) (9.1497, 19.7993) (9.6091, 21.4019) (9.8773, 22.671) (9.94, 23.2943) (9.9707, 23.5986) knots 0 0 0 0 0.062347 0.127633 0.196641 0.270049 0.348203 0.431234 0.519115 0.611423 0.806629 1.009594 1.210352 1.306485 1.398176 1.398176 1.398176 1.398176
  line L1870 (11, 25) -> (-11, 25)
  spline S78 degree 3 poles (-8.5, 10) (-8.6005, 9.7839) (-8.8038, 9.3472) (-9.1787, 8.7173) (-9.5868, 8.086) (-10.0277, 7.4531) (-10.4974, 6.8235) (-11.1586, 6.0064) (-11.6642, 5.4016) (-12, 5) knots 0 0 0 0 0.071451 0.144434 0.219638 0.296973 0.375788 0.45523 0.612272 0.612272 0.612272 0.612272
  spline S79 degree 3 poles (8.5, 10) (8.6005, 9.7839) (8.8038, 9.3472) (9.1787, 8.7173) (9.5868, 8.086) (10.0277, 7.4531) (10.4974, 6.8235) (11.1586, 6.0064) (11.6642, 5.4016) (12, 5) knots 0 0 0 0 0.071451 0.144434 0.219638 0.296973 0.375788 0.45523 0.612272 0.612272 0.612272 0.612272
  spline S80 degree 3 poles (-12, 5) (-12.1435, 4.8154) (-12.3572, 4.5405) (-12.6129, 4.1571) (-12.7867, 3.8671) (-12.9422, 3.5716) (-13.0787, 3.2704) (-13.195, 2.9629) (-13.2913, 2.6494) (-13.3686, 2.3302) (-13.4471, 1.8962) (-13.5027, 1.3423) (-13.5191, 0.6723) (-13.517, 0.224) (-13.516, 0) knots 0 0 0 0 0.070131 0.104405 0.138173 0.17151 0.20452 0.237328 0.270066 0.302853 0.33579 0.402309 0.469592 0.53679 0.53679 0.53679 0.53679
  spline S81 degree 3 poles (12, 5) (12.1435, 4.8154) (12.3572, 4.5405) (12.6129, 4.1571) (12.7867, 3.8671) (12.9422, 3.5716) (13.0787, 3.2704) (13.195, 2.9629) (13.2913, 2.6494) (13.3686, 2.3302) (13.4471, 1.8962) (13.5027, 1.3423) (13.5191, 0.6723) (13.517, 0.224) (13.516, 0) knots 0 0 0 0 0.070131 0.104405 0.138173 0.17151 0.20452 0.237328 0.270066 0.302853 0.33579 0.402309 0.469592 0.53679 0.53679 0.53679 0.53679
  spline S82 degree 3 poles (-11, 23.984) (-10.9832, 23.667) (-10.9477, 22.9996) (-10.7349, 21.978) (-10.4553, 20.9044) (-10.0046, 19.4423) (-9.5118, 18.0008) (-9.042, 16.593) (-8.7295, 15.606) (-8.4679, 14.6801) (-8.2663, 13.822) (-8.1301, 13.0341) (-8.0666, 12.3149) (-8.0765, 11.6602) (-8.1553, 11.0629) (-8.2957, 10.5116) (-8.4325, 10.1689) (-8.5, 10) knots 0 0 0 0 0.095122 0.200216 0.312183 0.428034 0.659064 0.769198 0.873257 0.96964 1.057768 1.137592 1.209313 1.274064 1.333591 1.389675 1.444205 1.444205 1.444205 1.444205
  spline S83 degree 3 poles (11, 23.984) (10.9832, 23.667) (10.9477, 22.9996) (10.7349, 21.978) (10.4553, 20.9044) (10.0046, 19.4423) (9.5118, 18.0008) (9.042, 16.593) (8.7295, 15.606) (8.4679, 14.6801) (8.2663, 13.822) (8.1301, 13.0341) (8.0666, 12.3149) (8.0765, 11.6602) (8.1553, 11.0629) (8.2957, 10.5116) (8.4325, 10.1689) (8.5, 10) knots 0 0 0 0 0.095122 0.200216 0.312183 0.428034 0.659064 0.769198 0.873257 0.96964 1.057768 1.137592 1.209313 1.274064 1.333591 1.389675 1.444205 1.444205 1.444205 1.444205
  line L1871 (-11, 23.984) -> (-11, 25)
  line L1872 (11, 23.984) -> (11, 25)
  line L1873 (8, -118.9769) -> (5.0731, -118.9769)
  line L1874 (2.82, -118.9769) -> (-7.8805, -118.9769)
  spline S84 degree 3 poles (-13.016, -93.9769) (-13.0152, -94.8292) (-13.014, -96.1053) (-12.9132, -97.8013) (-12.7748, -99.0629) (-12.5647, -100.3144) (-12.2783, -101.5542) (-11.9231, -102.7836) (-11.6374, -103.59) (-11.494, -103.9948) knots 0 0 0 0 0.25561 0.382747 0.509496 0.636178 0.763224 0.891032 1.019834 1.019834 1.019834 1.019834
  spline S85 degree 3 poles (13.016, -93.9769) (13.0115, -95.0469) (13.0047, -96.6486) (12.8212, -98.7741) (12.5626, -100.3493) (12.1857, -101.9056) (11.5434, -103.9672) (10.508, -106.4769) (9.4726, -108.9866) (8.8303, -111.0482) (8.4534, -112.6045) (8.1948, -114.1797) (8.0113, -116.3052) (8.0045, -117.9069) (8, -118.9769) knots 0 0 0 0 0.320849 0.480281 0.639462 0.799243 0.960292 1.286737 1.613182 1.774231 1.934012 2.093192 2.252625 2.573474 2.573474 2.573474 2.573474
  line L1875 (5, -89.9769) -> (5, -118.9769)
  line L1876 (-5, -89.9769) -> (-5, -118.9769)
  line L1877 (4.963, -89.9769) -> (4.963, -92.4769)
  line L1878 (3.185, -89.9769) -> (3.185, -92.4769)
  line L1879 (5.709, -89.9769) -> (5.709, -92.4769)
  line L1880 (3.931, -89.9769) -> (3.931, -92.4769)
  line L1881 (-8.605, -89.9769) -> (-8.605, -92.4769)
  line L1882 (-10.383, -89.9769) -> (-10.383, -92.4769)
  line L1883 (-12, -89.9769) -> (-12, -29.9769)
  line L1884 (12, -89.9769) -> (12, -29.9769)
  line L1885 (-13.016, -93.9769) -> (-13.016, -29.9769)
  line L1886 (13.016, -93.9769) -> (13.016, -29.9769)
  spline S86 degree 3 poles (-12, -29.9769) (-12.0003, -29.7681) (-12.001, -29.3509) (-12.039, -28.7256) (-12.1259, -28.1043) (-12.25, -27.4885) (-12.3741, -26.8726) (-12.461, -26.2513) (-12.499, -25.626) (-12.4997, -25.2088) (-12.5, -25) knots 0 0 0 0 0.062631 0.12514 0.187761 0.250672 0.313584 0.376205 0.438713 0.501345 0.501345 0.501345 0.501345
  spline S87 degree 3 poles (12, -29.9769) (12.0003, -29.7681) (12.001, -29.3509) (12.039, -28.7256) (12.1259, -28.1043) (12.25, -27.4885) (12.3741, -26.8726) (12.461, -26.2513) (12.499, -25.626) (12.4997, -25.2088) (12.5, -25) knots 0 0 0 0 0.062631 0.12514 0.187761 0.250672 0.313584 0.376205 0.438713 0.501345 0.501345 0.501345 0.501345
  spline S88 degree 3 poles (-13.516, -25) (-13.5157, -25.2088) (-13.515, -25.626) (-13.477, -26.2513) (-13.3901, -26.8726) (-13.266, -27.4885) (-13.1419, -28.1043) (-13.055, -28.7256) (-13.017, -29.3509) (-13.0163, -29.7681) (-13.016, -29.9769) knots 0 0 0 0 0.062631 0.12514 0.187761 0.250672 0.313584 0.376205 0.438713 0.501345 0.501345 0.501345 0.501345
  spline S89 degree 3 poles (13.516, -25) (13.5157, -25.2088) (13.515, -25.626) (13.477, -26.2513) (13.3901, -26.8726) (13.266, -27.4885) (13.1419, -28.1043) (13.055, -28.7256) (13.017, -29.3509) (13.0163, -29.7681) (13.016, -29.9769) knots 0 0 0 0 0.062631 0.12514 0.187761 0.250672 0.313584 0.376205 0.438713 0.501345 0.501345 0.501345 0.501345
  line L1887 (-12.5, -25) -> (-12.5, 0)
  line L1888 (12.5, -25) -> (12.5, 0)
  line L1889 (-13.516, -25) -> (-13.516, 0)
  line L1890 (13.516, -25) -> (13.516, 0)
  point P0 (0, 0)
  constraints: 4 end point, 1 parallel, 1 vertical, 2 other
sketch "Sketch14" plane through (0, 0, 0) normal (1, 0, 0) x (0, 1, 0)
  line L0 (-13.762, -15) -> (-13.762, 0) projected
  line L1 (13.762, 0) -> (-13.762, 0) projected
  line L2 (13.762, -15) -> (13.762, 0) projected
  line L3 (13, 0) -> (13, -15) projected
  line L4 (-13, 0) -> (-13, -15) projected
  line L5 (-13, 33) -> (5.5, 33)
  line L6 (5.5, 33) -> (5.5, 0)
  line L7 (5.5, 0) -> (-7.5, 0)
  line L8 (0, -156.7871) -> (0, 91.8442) projected
  line L9 (-5.5, 31.984) -> (5.5, 31.984)
  line L10 (-5.5, 31.984) -> (-5.5, 33)
  line L11 (-13.762, 0) -> (-13, 0)
  line L12 (0, 33) -> (0, 31.984)
  spline S0 degree 4 poles (-5.5, 31.984) (-8.299, 31.984) (-14.8344, 28.6033) (-3.4332, 19.5919) (-10.8112, 9.333) (-13, 3.9122) (-13, 0) knots 0 0 0 0 0 0.349131 0.599131 1 1 1 1 1
  spline S1 degree 4 poles (-5.5, 33) (-8.7004, 33) (-16.1149, 29.0043) (-4.4472, 20.0629) (-11.8632, 9.424) (-13.762, 3.8966) (-13.762, 0) knots 0 0 0 0 0 0.357205 0.607205 1 1 1 1 1
  point P0 (0, 0)
  point P1 (0, 0)
  point P2 (-10.8475, 28.6822)
  point P3 (-8.5755, 20.4298)
  point P4 (-10.1946, 9.9764)
  point P5 (-11.8109, 29.0047)
  point P6 (-9.5915, 20.5086)
  point P7 (-11.2106, 9.988)
  dimension "d94" = 33
  dimension "d95" = 1.016
  dimension "d96" = 11
  dimension "d203" = 1.016
  dimension "d204" = 1.016
  dimension "d205" = 1.016
  constraints: 14 end point, 5 point on line, 3 horizontal, 2 collinear, 2 midpoint, 2 parallel, 2 perpendicular, 2 vertical, 2 vertical alignment, 10 other
  measures "d94" distance between parallel lines of L1 L5
  measures "d95" distance between parallel lines of L9 L5
  measures "d96" distance between parallel lines of L6 L10
  measures "d203" distance of point (-10.847, 28.682) point (-11.811, 29.005)
  measures "d204" horizontal distance of point (-10.195, 9.976) point (-11.211, 9.988)
  measures "d205" horizontal distance of point (-8.576, 20.43) point (-9.592, 20.509)
revolve "Head" add sketch "Sketch14" angle 360 about axis through (0, 0, -10) along (0, 0, 1) contours L1 S1 L10 S0 | L10 L5 L8 L9
ref_plane "Work Plane8" through (0, 0, -94.9769) normal (0, 0, 1) x (1, 0, 0)
ref_plane "Work Plane9" through (0, 0, -68.9769) normal (0, 0, 1) x (1, 0, 0)
sketch "Sketch15" plane through (0, 0, -94.9769) normal (0, 0, 1) x (1, 0, 0)
  circle A0 centre (-8.737, 4.074) radius 0.889
  circle A1 centre (8.349, 4.82) radius 0.889
  circle A2 centre (0, -9.494) radius 0.889
  line L0 (-9.8917, 2.074) -> (-7.5823, 2.074)
  line L1 (-11.0464, 4.074) -> (-9.8917, 2.074)
  line L2 (-7.5823, 2.074) -> (-6.4276, 4.074)
  line L3 (-9.8917, 6.074) -> (-11.0464, 4.074)
  line L4 (-7.5823, 6.074) -> (-9.8917, 6.074)
  line L5 (-6.4276, 4.074) -> (-7.5823, 6.074)
  line L6 (1.1547, -7.494) -> (-1.1547, -7.494)
  line L7 (2.3094, -9.494) -> (1.1547, -7.494)
  line L8 (1.1547, -11.494) -> (2.3094, -9.494)
  line L9 (-1.1547, -11.494) -> (1.1547, -11.494)
  line L10 (-2.3094, -9.494) -> (-1.1547, -11.494)
  line L11 (-1.1547, -7.494) -> (-2.3094, -9.494)
  line L12 (7.1943, 6.82) -> (6.0396, 4.82)
  line L13 (9.5037, 6.82) -> (7.1943, 6.82)
  line L14 (10.6584, 4.82) -> (9.5037, 6.82)
  line L15 (9.5037, 2.82) -> (10.6584, 4.82)
  line L16 (7.1943, 2.82) -> (9.5037, 2.82)
  line L17 (6.0396, 4.82) -> (7.1943, 2.82)
  point P0 (0, 0)
  point P1 (0, 0)
  constraints: 36 end point, 3 centre point
hole "Hole3" at (0, -9.494, -94.9769) at (-8.737, 4.074, -94.9769) at (8.349, 4.82, -94.9769) direction (0, 0, 1) diameter 6 depth 26
ref_plane "Work Plane10" through (0, 13.762, -7.5) normal (0, 1, 0) x (-1, 0, 0)
sketch "Sketch16" plane through (0, 13.762, -7.5) normal (0, 1, 0) x (-1, 0, 0)
  line L0 (13.016, -22.4769) -> (-13.016, -22.4769) projected
  line L1 (-13.016, -61.4769) -> (-13.016, -22.4769) projected
  line L2 (0, -149.2871) -> (0, 99.3442) projected
  line L3 (0, -22.4769) -> (0, -7.5) projected
  line L4 (13.762, -7.5) -> (-13.762, -7.5) projected
  line L5 (13.016, -22.4769) -> (-13.016, -22.4769) projected
  line L6 (0, -7.5) -> (0, -22.4769) projected
  line L7 (-13.762, -7.5) -> (-13.762, 7.5) projected
  line L8 (13.762, -7.5) -> (13.762, 7.5) projected
  line L9 (-13, 7.5) -> (-13, -7.5) projected
  line L10 (13, 7.5) -> (13, -7.5) projected
  line L11 (-19.2668, -57.4769) -> (19.2668, -57.4769) projected
  line L12 (5.5, 40.5) -> (-5.5, 40.5) projected
  line L13 (-11, 9.5) -> (11, 9.5)
  line L14 (11, 9.5) -> (11, 7.5)
  line L15 (11, 7.5) -> (-11, 7.5)
  line L16 (-11, 7.5) -> (-11, 9.5)
  line L17 (-11, 7.5) -> (11, 7.5)
  line L18 (11, 7.5) -> (11, -7.5)
  line L19 (11, -7.5) -> (-11, -7.5)
  line L20 (-11, -7.5) -> (-11, 7.5)
  line L21 (-11, -7.5) -> (11, -7.5)
  line L22 (11, -7.5) -> (11, -22.4769)
  line L23 (11, -22.4769) -> (-11, -22.4769)
  line L24 (-11, -22.4769) -> (-11, -7.5)
  line L25 (-11, -22.4769) -> (11, -22.4769)
  line L26 (11, -22.4769) -> (11, -32.4769)
  line L27 (11, -32.4769) -> (-11, -32.4769)
  line L28 (-11, -32.4769) -> (-11, -22.4769)
  line L29 (-9.984, 8.484) -> (9.984, 8.484)
  line L30 (9.984, 8.484) -> (9.984, 7.5)
  line L31 (9.984, 7.5) -> (-9.984, 7.5)
  line L32 (-9.984, 7.5) -> (-9.984, 8.484)
  line L33 (-9.984, 7.5) -> (9.984, 7.5)
  line L34 (9.984, 7.5) -> (9.984, -7.5)
  line L35 (9.984, -7.5) -> (-9.984, -7.5)
  line L36 (-9.984, -7.5) -> (-9.984, 7.5)
  line L37 (-9.984, -7.5) -> (9.984, -7.5)
  line L38 (9.984, -7.5) -> (9.984, -22.4769)
  line L39 (9.984, -22.4769) -> (-9.984, -22.4769)
  line L40 (-9.984, -22.4769) -> (-9.984, -7.5)
  line L41 (-9.984, -22.4769) -> (9.984, -22.4769)
  line L42 (8.976, -32.4769) -> (-8.976, -32.4769)
  line L43 (-9.984, -22.4769) -> (9.984, -22.4769)
  line L44 (9.984, -22.4769) -> (9.984, -31.4609)
  line L45 (9.984, -31.4609) -> (-9.984, -31.4609)
  line L46 (-9.984, -31.4609) -> (-9.984, -22.4769)
  line L47 (13.762, 7.5) -> (-13.762, 7.5) projected
  point P0 (0, 7.5)
  point P1 (0, 40.5)
  point P2 (0, -7.5)
  point P3 (0, 9.5)
  point P4 (0, 7.5)
  point P5 (0, 7.5)
  point P6 (0, 8.484)
  point P7 (3.0653, 35.3698)
  dimension "d112" = 22
  dimension "d127" = 10
  dimension "d129" = 1.016
  dimension "d130" = 1.016
  dimension "d131" = 1.016
  dimension "d206" = 2
  constraints: 68 end point, 17 parallel, 9 coincident, 9 horizontal, 8 perpendicular, 6 midpoint, 6 point on line, 2 vertical alignment, 1 other
  measures "d112" distance between parallel lines of L14 L16
  measures "d127" distance between parallel lines of L27 L23
  measures "d129" distance between parallel lines of L32 L16
  measures "d130" distance between parallel lines of L42 L45
  measures "d131" distance between parallel lines of L29 L13
  measures "d206" distance between parallel lines of L15 L13
extrude "Extrusion4" add sketch "Sketch16" against normal up to next contours L15 L30 L29 L2 L13 L14 | L15 L2 L29 L30 | L15 L32 L29 L2 | L2 L29 L32 L15 L16 L13
extrude "Extrusion8" add sketch "Sketch16" against normal up to surface contours L4 L34 L15 L18 | L4 L2 L15 L34 | L4 L36 L15 L2 | L4 L20 L15 L36
extrude "Extrusion6" add sketch "Sketch16" against normal up to next contours L0 L38 L4 L22 | L0 L2 L4 L38 | L0 L40 L4 L2 | L0 L24 L4 L40
extrude "Extrusion7" add sketch "Sketch16" against normal up to surface contours L26 L27 L2 L45 L44 L0 | L44 L45 L2 L0 | L2 L45 L46 L0 | L46 L45 L2 L27 L28 L0
extrude "Extrusion9" cut sketch "Sketch16" against normal up to next contours L15 L2 L29 L30 | L15 L32 L29 L2
extrude "Extrusion10" cut sketch "Sketch16" against normal up to surface contours L4 L2 L15 L34 | L4 L36 L15 L2
extrude "Extrusion11" cut sketch "Sketch16" against normal blind 10 contours L0 L2 L4 L38 | L0 L40 L4 L2
extrude "Extrusion12" cut sketch "Sketch16" against normal up to surface contours L44 L45 L2 L0 | L2 L45 L46 L0